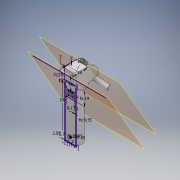
# Autodesk Inventor part: QC25BTFication_3
Saved by Autodesk Inventor 2018 (Build 220112000, 112)
## iProperties
Created: 2021-09-19
Part Number: QC25BTFication_3
Material: Generic
Document SubType Name: Modeling
Designer: dangl
Density: 1 g/cm^3
Appearance: Default
Author: dangl
Autodesk Inventor part; units mm, degrees
ref_plane "YZ Plane" through (0, 0, 0) normal (1, 0, 0) x (0, 1, 0)
ref_plane "XZ Plane" through (0, 0, 0) normal (0, 1, 0) x (-1, 0, 0)
ref_plane "XY Plane" through (0, 0, 0) normal (0, 0, 1) x (1, 0, 0)
sketch "Sketch3" plane through (0, 0, 0) normal (0, 1, 0) x (-1, 0, 0)
  line L0 (0, 0) -> (11, 0)
  line L1 (11, 0) -> (11, -56)
  line L2 (11, -56) -> (0, -56)
  line L3 (0, -56) -> (0, 0)
  line L4 (12, 1) -> (-1, 1)
  line L5 (-1, 1) -> (-1, -57)
  line L6 (-1, -57) -> (12, -57)
  line L7 (12, -57) -> (12, 1)
  line L8 (7.55, -6.2) -> (3.45, -6.2)
  line L9 (1.45, -8.2) -> (1.45, -12)
  line L10 (3.45, -14) -> (7.55, -14)
  line L11 (9.55, -12) -> (9.55, -8.2)
  arc A0 (9.55, -8.2) -> (7.55, -6.2) centre (7.55, -8.2) ccw
  arc A1 (7.55, -14) -> (9.55, -12) centre (7.55, -12) ccw
  arc A2 (1.45, -12) -> (3.45, -14) centre (3.45, -12) ccw
  arc A3 (3.45, -6.2) -> (1.45, -8.2) centre (3.45, -8.2) ccw
  circle A4 centre (5.5, -51) radius 1
  point P0 (1.45, -14)
  point P1 (1.45, -6.2)
  point P2 (9.55, -14)
  dimension "d2" = 11
  dimension "d3" = 56
  dimension "d4" = 1
  dimension "d5" = 1
  dimension "d6" = 1
  dimension "d7" = 1
  dimension "d8" = 8.1
  dimension "d9" = 7.8
  dimension "d10" = 14
  dimension "d11" = 9.55
  dimension "d12" = 2
  dimension "d30" = 2
  dimension "d31" = 5
  dimension "d32" = 5.5
  constraints: 24 end point, 8 point on circle, 8 tangent, 6 parallel, 6 point on line, 5 centre point, 3 equal radius, 3 horizontal, 3 perpendicular
  measures "d2" distance of L1.end L2.end
  measures "d3" distance of L0.end L1.end
  measures "d4" distance between parallel lines of L1 L7
  measures "d5" distance between parallel lines of L2 L6
  measures "d6" distance between parallel lines of L0 L4
  measures "d7" distance between parallel lines of L5 L3
  measures "d8" distance of point (1.45, -14) point (9.55, -14)
  measures "d9" distance of point (1.45, -6.2) point (1.45, -14)
  measures "d10" distance between parallel lines of L0 L10
  measures "d11" distance between parallel lines of L3 L11
  measures "d12" radius of A0
  measures "d30" diameter of A4
  measures "d31" distance from line of L2 A4.centre
  measures "d32" distance from line of L3 A4.centre
extrude "Extrusion1" add sketch "Sketch3" along normal blind 1.4 contours L0 L1 L2 L3
extrude "Extrusion3" add sketch "Sketch3" along normal blind 8.6 contours L7 L6 L5 L4
sketch "Sketch4" plane through (-12, 0, 1) normal (0, 0, 1) x (1, 0, 0)
  circle A0 centre (6.5, 5.4) radius 2.65
  line L0 (0, 0) -> (0, 8.6) projected
  line L1 (0, 0) -> (13, 0) projected
  point P0 (12, 0)
  dimension "d19" = 6.5
  dimension "d20" = 5.3
  dimension "d21" = 5.4
  constraints: 1 centre point
  measures "d19" distance from line of L0 A0.centre
  measures "d20" diameter of A0
  measures "d21" distance from line of L1 A0.centre
extrude "Extrusion4" cut sketch "Sketch4" against normal blind 8.6
sketch "Sketch5" plane through (1, 0, -57) normal (0, 0, -1) x (-1, 0, 0)
  line L0 (2.675, 6.25) -> (10.325, 6.25)
  line L1 (10.325, 6.25) -> (10.325, 3.55)
  line L2 (10.325, 3.55) -> (2.675, 3.55)
  line L3 (2.675, 3.55) -> (2.675, 6.25)
  line L4 (0, 0) -> (13, 0) projected
  line L5 (13, 0) -> (13, 8.6) projected
  point P0 (1, 0)
  dimension "d24" = 7.65
  dimension "d25" = 2.7
  dimension "d26" = 3.55
  dimension "d27" = 2.675
  constraints: 8 end point, 2 parallel, 1 horizontal, 1 perpendicular
  measures "d24" distance of L0.start L0.end
  measures "d25" distance of L0.end L1.end
  measures "d26" distance between parallel lines of L4 L2
  measures "d27" distance between parallel lines of L5 L1
extrude "Extrusion5" cut sketch "Sketch5" against normal blind 8.6
sketch "Sketch6" plane through (0, 0, 0) normal (0, 1, 0) x (-1, 0, 0)
  line L0 (46.884994, 6) -> (-33.715052, 6)
  line L1 (12, 1) -> (-1, 1)
  point P0 (0, 0)
  dimension "d33" = 5
  constraints: 2 end point, 1 horizontal
  measures "d33" distance between parallel lines of L1 L0
ref_plane "Work Plane1" through (-46.884994, 0, 6) normal (0, -0.8660254, -0.5) x (1, 0, 0)
ref_plane "Work Plane2" through (-46.884994, 12.990381, 13.5) normal (0, -0.8660254, -0.5) x (1, 0, 0)
sketch "Sketch8" plane through (-46.884994, 12.990381, 13.5) normal (0, -0.8660254, -0.5) x (1, 0, 0)
  line L0 (41.384994, -17.002165) -> (59.239153, -23.500548)
  line L1 (47.884994, -8.630127) -> (47.884994, -58.8596)
  line L2 (34.884994, -4.330127) -> (47.884994, -4.330127)
  line L3 (46.884994, -57.993575) -> (46.884994, -9.496152)
  line L4 (59.239153, -23.500548) -> (60.333618, -20.493532)
  line L5 (60.333618, -20.493532) -> (42.479458, -13.995149)
  line L6 (42.479458, -13.995149) -> (41.384994, -17.002165)
  point P0 (46.884994, -5.196152)
  dimension "d42" = 70
  dimension "d44" = 5.5
  dimension "d45" = 19
  dimension "d46" = 3.2
  constraints: 8 end point, 2 perpendicular, 1 parallel
  measures "d42" angle of L0 L1
  measures "d44" distance from line of L3 L0.start
  measures "d45" distance of L0.start L0.end
  measures "d46" distance of L0.end L4.end
revolve "Revolution1" add sketch "Sketch8" angle 360 about axis through (-5.5, 21.491464, -1.224307) along (0.9396926, 0.1710101, -0.2961981)
sketch "Sketch11" plane through (0, 0, 0) normal (1, 0, 0) x (0, 1, 0)
  line L0 (17.18469, -15.453857) -> (-9.272315, -15.453857)
  line L1 (-9.272315, -15.453857) -> (-9.272315, -62.433582)
  line L2 (-9.272315, -62.433582) -> (17.18469, -62.433582)
  line L3 (17.18469, -62.433582) -> (17.18469, -15.453857)
  point P0 (0, 0)
  constraints: 8 end point, 2 parallel, 1 horizontal, 1 perpendicular
extrude "Extrusion8" [suppressed]
sketch "Sketch12" plane through (1, 0, 1) normal (1, 0, 0) x (0, 0, -1)
  line L0 (1.625326, 24.6) -> (3.5, 13.1)
  line L1 (3.5, 13.1) -> (5.5, 13.1)
  line L2 (5.5, 13.1) -> (6.253809, 9.682139)
  line L3 (6.253809, 9.682139) -> (12.155416, 8.6)
  line L4 (1, 8.6) -> (16.453857, 8.6)
  line L5 (0, 8.6) -> (12.155416, 8.6)
  line L6 (0, 8.6) -> (16.453857, 8.6)
  line L7 (1.625326, 24.6) -> (0, 24.6)
  line L8 (0, 24.6) -> (0, 8.6)
  point P0 (1, 0)
  dimension "d54" = 2
  dimension "d55" = 3.5
  dimension "d56" = 4.5
  dimension "d57" = 6
  dimension "d59" = 16
  constraints: 18 end point, 1 point on line
  measures "d54" distance of L0.end L1.end
  measures "d55" distance of L1.end L2.end
  measures "d56" distance between parallel lines of L4 L1
  measures "d57" distance of L2.end L3.end
  measures "d59" distance between parallel lines of L4 L7
extrude "Extrusion9" add sketch "Sketch12" against normal blind 1
sketch "Sketch13" plane through (-12, 0, 1) normal (-1, 0, 0) x (0, 0, 1)
  line L0 (0, 8.6) -> (0, 24.6)
  line L1 (0, 8.6) -> (-12.155416, 8.6)
  line L2 (0, 8.6) -> (-16, 8.6)
  line L3 (-58, 8.6) -> (0, 8.6)
  line L4 (-16, 8.6) -> (0, 24.6)
  line L5 (0, 0) -> (-58, 0)
  line L6 (0, 0) -> (10.5, 0)
  line L7 (12.5, 2) -> (12.5, 12.1)
  line L8 (0, 24.6) -> (0, 24.6)
  line L9 (0, 8.6) -> (0, 2)
  line L10 (-1, 1.4) -> (-1, 8.6)
  arc A0 (10.5, 0) -> (12.5, 2) centre (10.5, 2) ccw
  arc A1 (12.5, 12.1) -> (0, 24.6) centre (0, 12.1) ccw
  line L11 (0, 0) -> (0, 8.6)
  line L12 (0, 2) -> (10.5, 2)
  line L13 (10.5, 2) -> (10.5, 12.1)
  line L14 (0, 2) -> (0, 0)
  line L15 (10.5, 12.1) -> (12.5, 12.1)
  point P0 (-1, 0)
  point P1 (-16.453857, 8.6)
  point P2 (-16.453857, 0)
  point P3 (12.5, 0)
  dimension "d66" = 16
  dimension "d67" = 16
  dimension "d77" = 12.5
  dimension "d78" = 2
  dimension "d79" = 12.5
  dimension "d94" = 2
  dimension "d95" = 2
  constraints: 22 end point, 4 point on circle, 4 point on line, 4 tangent, 3 horizontal, 2 centre point, 2 parallel, 2 perpendicular, 2 vertical
  measures "d66" distance of L0.start L0.end
  measures "d67" distance of L0.start L2.end
  measures "d77" distance of L5.start point (12.5, 0)
  measures "d78" radius of A0
  measures "d79" radius of A1
  measures "d94" distance between parallel lines of L7 L13
  measures "d95" distance between parallel lines of L6 L12
extrude "Extrusion11" add sketch "Sketch13" against normal blind 1 contours L1 L2 L4 L0
sketch "Sketch14" plane through (12.35416, 24.740655, -6.852072) normal (0.9396926, 0.1710101, -0.2961981) x (-0.3006266, 0, -0.9537419)
  circle A0 centre (0, 0) radius 2
  line L0 (-2, 0) -> (-3.2, 0)
  line L1 (2, 0) -> (3.525, 0)
  line L2 (-3.2, 0) -> (-3.2, 4)
  arc A1 (-2.322138, 2.201743) -> (-1.433381, -2.861017) centre (0, 0) ccw
  line L3 (-3.2, 4) -> (3.525, 4)
  line L4 (3.525, 4) -> (3.525, 0)
  point P0 (-2.821119, -22.008984)
  dimension "d70" = 4
  dimension "d88" = 4
  constraints: 10 end point, 2 perpendicular, 2 point on circle, 1 centre point, 1 coincident, 1 horizontal, 1 point on line, 1 tangent, 1 vertical
  measures "d70" diameter of A0
  measures "d88" distance of L0.end L2.end
extrude "Extrusion12" cut sketch "Sketch14" against normal up to surface surface through (-11, 0, -56) normal (-1, 0, 0)
sketch "Sketch15" plane through (-5.5, 21.491464, -1.224307) normal (-0.9396926, -0.1710101, 0.2961981) x (0.3006266, 0, 0.9537419)
  arc A0 (-3.2, 0) -> (3.2, 0) centre (0, 0) ccw projected
  line L0 (3.2, 0) -> (2, 0) projected
  arc A1 (-2, 0) -> (2, 0) centre (0, 0) ccw projected
  line L1 (-2, 0) -> (-3.2, 0) projected
  point P0 (2.821119, -22.008984)
extrude "Extrusion13" add sketch "Sketch15" along normal up to surface surface through (-11, 0, -56) normal (-1, 0, 0)
sketch "Sketch16" plane through (-12, 0, 1) normal (0, 0, 1) x (1, 0, 0)
  line L0 (1, 17.252017) -> (1, 8.6)
  line L1 (1, 8.6) -> (1, 5.4)
  line L2 (1, 5.4) -> (3.85, 5.4)
  circle A0 centre (6.5, 5.4) radius 2.65
  line L3 (1, 8.6) -> (12, 8.6)
  line L4 (1, 8.6) -> (12, 8.6)
  line L5 (12, 8.6) -> (12, 5.4)
  line L6 (12, 8.6) -> (12, 1.4)
  line L7 (3.85, 5.4) -> (12, 5.4)
  point P0 (12, 0)
  constraints: 10 end point, 2 perpendicular, 2 point on line, 1 collinear, 1 horizontal alignment, 1 vertical, 1 other
extrude "Extrusion14" cut sketch "Sketch16" against normal blind 1.25 contours L3 L5 L7 A0 L2 L1 | A0 L7 picked at (7.236697, 6.607659)
extrude "Extrusion16" add sketch "Sketch13" against normal blind 1.5 contours L12 L13 L15 L7 A0 L6 L11
sketch "Sketch17" plane through (1, 0, 1) normal (1, 0, 0) x (0, 0, -1)
  line L0 (0, 8.6) -> (0, 24.6) projected
  line L1 (0, 0) -> (0, 8.6) projected
  line L2 (58, 0) -> (-10.5, 0) projected
  arc A0 (-12.5, 2) -> (-10.5, 0) centre (-10.5, 2) ccw projected
  line L3 (-12.5, 2) -> (-12.5, 12.1) projected
  arc A1 (0, 24.6) -> (-12.5, 12.1) centre (0, 12.1) ccw projected
  point P0 (1, 0)
  point P1 (16.453857, 0)
extrude "Extrusion17" add sketch "Sketch17" against normal blind 1.5
extrude "Extrusion18" add sketch "Sketch13" against normal up to surface (11.5 mm away) contours L12 L13 L15 L7 A0 L6 L11
extrude "Extrusion20" add sketch "Sketch13" against normal blind 2 contours L0 A1 L15 L13 L12 L9
equation "\"d11\" = 0.5 * d2 + 0.5 * d8"
equation "\"d32\" = 0.5 * d2"
equation "\"d19\" = 0.5 * d2 + d4"
equation "\"d44\" = 0.5 * d2"
equation "\"d60\" = d7"
equation "\"d68\" = d4"
equation "\"d88\" = d70"
body "Solid1"
